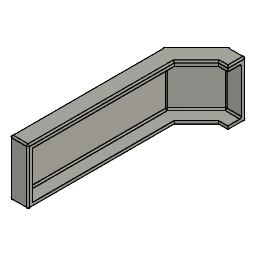
case left v13 (Autodesk Fusion 360 design; units mm, degrees)
Autodesk Fusion 360 part; units mm, degrees
sketch "Sketch1" plane through (0, 0, 0) normal (0, 0, 1) x (1, 0, 0)
  line L0 (0, 0) -> (0, 98) construction
  line L1 (0, 98) -> (20, 118) construction
  line L2 (20, 118) -> (30, 118) construction
  line L3 (9, 0) -> (9, 94.2721)
  line L4 (9, 94.2721) -> (23.7279, 109)
  line L5 (23.7279, 109) -> (30, 109)
  line L6 (-3, 0) -> (-3, 99.2426)
  line L7 (-3, 99.2426) -> (18.7574, 121)
  line L8 (18.7574, 121) -> (30, 121)
  line L9 (0, 0) -> (9, 0) construction
  line L10 (0, 0) -> (-3, 0) construction
  line L11 (30, 118) -> (30, 109)
  line L12 (30, 118) -> (30, 121)
  line L13 (0, -3) -> (9, -3)
  line L14 (0, -3) -> (-3, -3)
  line L15 (9, -3) -> (9, 0)
  line L16 (-3, -3) -> (-3, 0)
  dimension "d7" = 98
  dimension "d8" = 135
  dimension "d9" = 118
  dimension "d10" = 10
  dimension "d11" = 9
  dimension "d12" = -3
  dimension "d13" = 3
  constraint coincident L0.start L9.start
  constraint vertical L0
  constraint perpendicular L0 L2
  constraint perpendicular L3 L9
  constraint perpendicular L6 L10
  constraint perpendicular L5 L11
  constraint perpendicular L8 L12
  constraint perpendicular L9 L15
  constraint perpendicular L10 L16
  measures "d7" distance of L0.start L0.end
  measures "d8" angle of L0 L1
  measures "d9" vertical distance of L0.start L1.end
  measures "d10" distance of L1.end L2.end
extrude "Extrude1" add sketch "Sketch1" along normal blind 37.22
shell "Shell1" thickness 3 removed faces 6 at (30, 119, 12.4067) at (30, 115, 24.8133) at (25.8186, 109, 12.4067) at (13.9093, 99.1814, 24.8133) at (9, -2, 12.4067) at (9, 31.424, 12.4067)
fillet "Fillet2" radius 1 2 edges at (25, 118, 34.22) (25, 118, 3) 8 faces at (0, 65.3333, 23.8133) (6.6667, 104.6667, 13.4067) (1, -3, 12.4067) (1, 63.5049, 37.22) (22.5049, 121, 12.4067) (4.2525, 106.4951, 12.4067) (1, 63.5049, 0) (-3, 31.0809, 12.4067)
